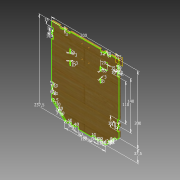
# Autodesk Inventor part: chassi_mdf
Saved by Autodesk Inventor 2014 (Build 180170000, 170)
## iProperties
Created: 2014-11-10
Part Number: chassi_mdf
Material: Generic
Document SubType Name: Modeling
Designer: Gabriel
Density: 1 g/cm^3
Appearance: Default
Author: Gabriel
Autodesk Inventor part; units mm, degrees
ref_plane "YZ Plane" through (0, 0, 0) normal (1, 0, 0) x (0, 1, 0)
ref_plane "XZ Plane" through (0, 0, 0) normal (0, 1, 0) x (-1, 0, 0)
ref_plane "XY Plane" through (0, 0, 0) normal (0, 0, 1) x (1, 0, 0)
sketch "Sketch1" plane through (0, 0, 0) normal (0, 1, 0) x (-1, 0, 0)
  line L0 (40, -237.5) -> (40, -237.5)
  line L1 (40, -237.5) -> (40, -237.5)
  line L2 (0, 0) -> (2.5, 0)
  line L3 (40, -237.5) -> (40, -237.5)
  line L4 (0, -90) -> (0, -80)
  line L5 (0, -70) -> (0, -45)
  line L6 (5, -45) -> (5, -35)
  line L7 (5, -35) -> (0, -35)
  line L8 (0, -35) -> (0, -25)
  line L9 (0, -25) -> (5, -25)
  line L10 (5, -25) -> (5, -15)
  line L11 (5, -15) -> (0, -15)
  line L12 (195, -45) -> (195, -35)
  line L13 (195, -35) -> (200, -35)
  line L14 (195, -25) -> (195, -15)
  line L15 (195, -15) -> (200, -15)
  line L16 (0, 0) -> (25, 0)
  line L17 (25, 0) -> (25, -5)
  line L18 (25, -5) -> (35, -5)
  line L19 (35, -5) -> (35, 0)
  line L20 (45, -5) -> (45, 0)
  line L21 (45, -5) -> (55, -5)
  line L22 (55, -5) -> (55, 0)
  line L23 (200, 0) -> (175, 0)
  line L24 (175, 0) -> (175, -5)
  line L25 (175, -5) -> (165, -5)
  line L26 (165, -5) -> (165, 0)
  line L27 (155, -5) -> (155, 0)
  line L28 (155, -5) -> (145, -5)
  line L29 (145, -5) -> (145, 0)
  line L30 (195, -45) -> (200, -45)
  line L31 (200, -45) -> (195, -45)
  line L32 (0, -45) -> (5, -45)
  line L33 (35, -35) -> (35, -25)
  line L34 (35, -45) -> (55, -45)
  line L35 (55, -45) -> (55, -43.5)
  line L36 (146.5, -45) -> (145, -45)
  line L37 (145, -45) -> (145, -43.5)
  line L38 (55, -85) -> (53.5, -85)
  line L39 (145, -85) -> (146.5, -85)
  line L40 (55, -85) -> (55, -75) construction
  line L41 (56.5, -85) -> (56.5, -75)
  line L42 (53.5, -75) -> (53.5, -85)
  arc A0 (53.5, -85) -> (56.5, -85) centre (55, -85) ccw
  arc A1 (56.5, -75) -> (53.5, -75) centre (55, -75) ccw
  line L43 (145, -85) -> (145, -75) construction
  line L44 (146.5, -85) -> (146.5, -75)
  line L45 (143.5, -75) -> (143.5, -85)
  arc A2 (143.5, -85) -> (146.5, -85) centre (145, -85) ccw
  arc A3 (146.5, -75) -> (143.5, -75) centre (145, -75) ccw
  line L46 (55, -45) -> (55, -55) construction
  line L47 (53.5, -45) -> (53.5, -55)
  line L48 (56.5, -55) -> (56.5, -45)
  arc A4 (56.5, -45) -> (53.5, -45) centre (55, -45) ccw
  arc A5 (53.5, -55) -> (56.5, -55) centre (55, -55) ccw
  line L49 (145, -45) -> (145, -55) construction
  line L50 (143.5, -45) -> (143.5, -55)
  line L51 (146.5, -55) -> (146.5, -45)
  arc A6 (146.5, -45) -> (143.5, -45) centre (145, -45) ccw
  arc A7 (143.5, -55) -> (146.5, -55) centre (145, -55) ccw
  line L52 (0, -185) -> (0, -200)
  line L53 (200, -187.5) -> (200, -200)
  line L54 (200, -187.5) -> (200, -200)
  circle A8 centre (2.5, -170) radius 1.5
  line L55 (0, -138.5) -> (0, -155)
  line L56 (2.5, -175) -> (0, -175)
  line L57 (0, -175) -> (5, -175)
  line L58 (5, -175) -> (5, -185)
  line L59 (5, -185) -> (0, -185)
  line L60 (2.5, -165) -> (0, -165)
  line L61 (2.5, -165) -> (5, -165)
  line L62 (5, -165) -> (5, -155)
  line L63 (5, -155) -> (0, -155)
  line L64 (0, -25) -> (5, -25)
  line L65 (195, -25) -> (200, -25)
  line L66 (0, -25) -> (5, -25)
  line L67 (35, -25) -> (40, -25)
  line L68 (2.5, -35) -> (2.5, -30)
  circle A9 centre (2.5, -30) radius 1.5
  line L69 (40, 0) -> (40, -2.5)
  circle A10 centre (40, -2.5) radius 1.5
  line L70 (160, -1) -> (160, -2.5)
  circle A11 centre (160, -2.5) radius 1.5
  line L71 (197.5, -35) -> (197.5, -30)
  circle A12 centre (197.5, -30) radius 1.5
  line L72 (200, -145) -> (200, -135)
  line L73 (200, -135) -> (200, -145)
  line L74 (200, -135) -> (200, -145)
  line L75 (200, -82.5) -> (200, -90)
  line L76 (200, -100) -> (200, -125)
  line L77 (200, -80) -> (200, -82.5)
  line L78 (200, -82.5) -> (200, -90)
  line L79 (200, -100) -> (200, -125)
  line L80 (0, -120) -> (0, -100)
  line L81 (0, -90) -> (0, -80)
  line L82 (0, -70) -> (0, 0)
  line L83 (0, -175) -> (0, -165)
  line L84 (0, -155) -> (0, -120)
  line L85 (80, -237.5) -> (120, -237.5)
  line L86 (0, 0) -> (25, 0)
  line L87 (35, 0) -> (45, 0)
  line L88 (55, 0) -> (145, 0)
  line L89 (155, 0) -> (165, 0)
  line L90 (175, 0) -> (200, 0)
  line L91 (200, 0) -> (200, -15)
  line L92 (200, -25) -> (200, -35)
  line L93 (200, -45) -> (200, -70)
  line L94 (0, -100) -> (0, -90)
  line L95 (0, -80) -> (0, -70)
  line L96 (200, -100) -> (200, -90)
  line L97 (200, -80) -> (200, -70)
  line L98 (0, -175) -> (0, -165)
  line L99 (0, -155) -> (0, -120)
  line L100 (0, -120) -> (0, -155)
  line L101 (0, -165) -> (0, -175)
  line L102 (0, -175) -> (0, -165)
  line L103 (0, -155) -> (0, -100)
  line L104 (200, -125) -> (200, -135)
  line L105 (200, -145) -> (200, -155)
  circle A13 centre (197.5, -170) radius 1.5
  line L106 (200, -170) -> (200, -165)
  line L107 (200, -165) -> (195, -165)
  line L108 (195, -165) -> (195, -155)
  line L109 (195, -155) -> (200, -155)
  line L110 (200, -170) -> (200, -175)
  line L111 (200, -175) -> (195, -175)
  line L112 (195, -175) -> (195, -185)
  line L113 (195, -185) -> (200, -185)
  line L114 (200, -165) -> (200, -175)
  line L115 (200, -185) -> (200, -187.5)
  line L116 (200, -165) -> (200, -175)
  line L117 (200, -185) -> (200, -187.5)
  line L118 (2.5, -170) -> (4, -170)
  line L119 (40, -237.5) -> (50, -237.5)
  line L120 (60, -237.5) -> (70, -237.5)
  line L121 (40, -237.5) -> (50, -237.5)
  line L122 (50, -237.5) -> (50, -232.5)
  line L123 (50, -232.5) -> (60, -232.5)
  line L124 (60, -232.5) -> (60, -237.5)
  line L125 (60, -237.5) -> (70, -237.5)
  line L126 (70, -237.5) -> (70, -232.5)
  line L127 (70, -232.5) -> (80, -232.5)
  line L128 (80, -232.5) -> (80, -237.5)
  circle A14 centre (65, -235) radius 1.5
  line L129 (160, -237.5) -> (150, -237.5)
  line L130 (150, -237.5) -> (150, -232.5)
  line L131 (150, -232.5) -> (140, -232.5)
  line L132 (140, -232.5) -> (140, -237.5)
  line L133 (140, -237.5) -> (130, -237.5)
  line L134 (130, -237.5) -> (130, -232.5)
  line L135 (130, -232.5) -> (120, -232.5)
  line L136 (120, -232.5) -> (120, -237.5)
  line L137 (130, -237.5) -> (140, -237.5)
  line L138 (150, -237.5) -> (160, -237.5)
  circle A15 centre (135, -235) radius 1.5
  line L139 (40, -237.5) -> (40, -232.5)
  line L140 (160, -237.5) -> (160, -232.5)
  line L141 (195, -204.6875) -> (191.0053, -208.4325)
  line L142 (191.0053, -208.4325) -> (195, -204.6875)
  line L143 (194.9237, -204.759) -> (200, -200)
  line L144 (160, -237.5) -> (169.1192, -228.9507)
  line L145 (169.1192, -228.9507) -> (165.6995, -225.303)
  line L146 (165.6995, -225.303) -> (172.9949, -218.4636)
  line L147 (172.9949, -218.4636) -> (176.4146, -222.1113)
  line L148 (180.2903, -211.6242) -> (183.71, -215.2719)
  line L149 (180.2903, -211.6242) -> (187.5856, -204.7848)
  line L150 (187.5856, -204.7848) -> (191.0053, -208.4325)
  line L151 (176.4146, -222.1113) -> (180.0623, -218.6916)
  line L152 (180.0623, -218.6916) -> (178.3524, -216.8678)
  circle A16 centre (178.3524, -216.8678) radius 1.5
  line L153 (160, -237.5) -> (169.1192, -228.9507)
  line L154 (176.4146, -222.1113) -> (183.71, -215.2719)
  line L155 (191.0053, -208.4325) -> (195, -204.6875)
  line L156 (40, -237.5) -> (30.8808, -228.9507)
  line L157 (30.8808, -228.9507) -> (34.3005, -225.303)
  line L158 (34.3005, -225.303) -> (27.0051, -218.4636)
  line L159 (27.0051, -218.4636) -> (23.5854, -222.1113)
  line L160 (19.7097, -211.6242) -> (16.29, -215.2719)
  line L161 (19.7097, -211.6242) -> (12.4144, -204.7848)
  line L162 (12.4144, -204.7848) -> (8.9947, -208.4325)
  line L163 (23.5854, -222.1113) -> (19.9377, -218.6916)
  line L164 (19.9377, -218.6916) -> (21.6476, -216.8678)
  circle A17 centre (21.6476, -216.8678) radius 1.5
  line L165 (8.9947, -208.4325) -> (0, -200)
  line L166 (40, -237.5) -> (30.8808, -228.9507)
  line L167 (23.5854, -222.1113) -> (16.29, -215.2719)
  line L168 (160, -237.5) -> (200, -200)
  line L169 (200, -200) -> (200, -195)
  line L170 (160, -237.5) -> (156.5803, -233.8523)
  line L171 (156.5803, -233.8523) -> (165.6995, -225.303)
  line L172 (187.5856, -204.7848) -> (196.7048, -196.2356)
  line L173 (196.7048, -196.2356) -> (200, -200)
  line L174 (160, -237.5) -> (160, -230.6463)
  line L175 (200, -200) -> (192.6894, -200)
  point P0 (55, -80)
  point P1 (145, -80)
  point P2 (55, -50)
  point P3 (145, -50)
  dimension "d489" = 3
  dimension "d514" = 3
  dimension "d41" = 2.5
  dimension "d381" = 5
  dimension "d382" = 10
  dimension "d383" = 10
  dimension "d384" = 5
  dimension "d385" = 10
  dimension "d392" = 5
  dimension "d393" = 10
  dimension "d458" = 35
  dimension "d460" = 20
  dimension "d465" = 10
  dimension "d466" = 3
  dimension "d467" = 10
  dimension "d468" = 3
  dimension "d469" = 10
  dimension "d470" = 3
  dimension "d471" = 10
  dimension "d472" = 3
  dimension "d512" = 3
  dimension "d513" = 3
  dimension "d515" = 3
  dimension "d530" = 10
  dimension "d531" = 5
  dimension "d532" = 5
  dimension "d533" = 10
  dimension "d535" = 200
  dimension "d573" = 10
  dimension "d574" = 140
  dimension "d575" = 110
  dimension "d576" = 30
  dimension "d580" = 15
  dimension "d581" = 3
  dimension "d583" = 5
  dimension "d584" = 10
  dimension "d586" = 5
  dimension "d587" = 10
  dimension "d594" = 120
  dimension "d595" = 10
  dimension "d596" = 5
  dimension "d597" = 10
  dimension "d598" = 10
  dimension "d599" = 10
  dimension "d600" = 3
  dimension "d602" = 5
  dimension "d603" = 10
  dimension "d604" = 10
  dimension "d605" = 10
  dimension "d606" = 3
  dimension "d611" = 40
  dimension "d612" = 25
  dimension "d613" = 70
  dimension "d636" = 200
  dimension "d637" = 37.5
  dimension "d638" = 237.5
  dimension "d653" = 5
  dimension "d654" = 10
  dimension "d655" = 10
  dimension "d656" = 10
  dimension "d657" = 5
  dimension "d658" = 2.5
  dimension "d659" = 3
  dimension "d662" = 5
  dimension "d663" = 90
  dimension "d664" = 10
  constraints: 360 end point, 158 perpendicular, 59 parallel, 20 collinear, 18 point on circle, 16 centre point, 16 tangent, 15 point on line, 11 midpoint, 7 coincident, 1 horizontal alignment, 1 vertical alignment, 4 other
  measures "d41" distance of L2.start L2.end
  measures "d381" distance of L6.start L5.end
  measures "d382" distance of L6.start L6.end
  measures "d383" distance of L7.end L8.end
  measures "d384" distance of L8.end L9.end
  measures "d385" distance of L9.end L10.end
  measures "d392" distance of L16.end L17.end
  measures "d393" distance of L17.end L18.end
  measures "d458" distance of L5.end L34.start
  measures "d460" distance of L34.start L34.end
  measures "d465" distance of L38.start L40.end
  measures "d466" diameter of A1
  measures "d467" distance of L39.start L43.end
  measures "d468" diameter of A3
  measures "d469" distance of L34.end L46.end
  measures "d470" diameter of A5
  measures "d471" distance of L36.end L49.end
  measures "d472" diameter of A7
  measures "d512" diameter of A9
  measures "d513" diameter of A10
  measures "d515" diameter of A12
  measures "d530" distance between parallel lines of L65 L15
  measures "d531" distance from line of L71.end L65
  measures "d532" distance from line of L13 L71.end
  measures "d533" distance from line of L30 L71.start
  measures "d535" distance of L52.end point (0, 0)
  measures "d573" distance of L56.start L60.start
  measures "d574" distance of L68.end L118.start
  measures "d575" distance between parallel lines of L32 L63
  measures "d576" distance between parallel lines of L59 L63
  measures "d580" distance between parallel lines of L23 L15
  measures "d581" diameter of A13
  measures "d583" distance of L106.end L107.end
  measures "d584" distance of L107.end L108.end
  measures "d586" distance of L110.end L111.end
  measures "d587" distance of L111.end L112.end
  measures "d594" distance of L129.start L0.end
  measures "d595" distance of L0.end L119.end
  measures "d596" distance of L119.end L122.end
  measures "d597" distance of L122.end L123.end
  measures "d598" distance of L120.start L120.end
  measures "d599" distance of L126.end L127.end
  measures "d600" diameter of A14
  measures "d602" distance of L129.end L130.end
  measures "d603" distance of L130.end L131.end
  measures "d604" distance of L132.end L133.end
  measures "d605" distance of L134.end L135.end
  measures "d606" diameter of A15
  measures "d611" distance between parallel lines of L136 L128
  measures "d612" horizontal distance of A14.centre L0.start
  measures "d613" distance of A15.centre A14.centre
  measures "d636" distance between parallel lines of L91 L82
  measures "d637" distance from line of L85 L52.end
  measures "d638" distance between parallel lines of L129 L88
  measures "d653" distance of L144.end L145.end
  measures "d654" distance of L145.end L146.end
  measures "d655" distance of L146.end L148.start
  measures "d656" distance of L148.start L149.end
  measures "d657" distance of L147.end L151.end
  measures "d658" distance of L151.end L152.end
  measures "d659" diameter of A16
  measures "d662" distance of L156.end L157.end
  measures "d663" angle of L156 L157
  measures "d664" distance of L157.end L158.end
ref_plane "Work Plane2" through (0, 0, 0) normal (0, -1, 0) x (1, 0, 0)
sketch "Sketch2" plane through (0, 0, 0) normal (0, -1, 0) x (1, 0, 0)
  line L0 (-100, -2.5) -> (-100, -12.5)
  line L1 (-100, -12.5) -> (-90, -12.5)
  line L2 (-100, -12.5) -> (-110, -12.5)
  circle A0 centre (-90, -12.5) radius 2.5
  circle A1 centre (-110, -12.5) radius 2.5
  line L3 (-90, -12.5) -> (-90, -52.5)
  line L4 (-90, -52.5) -> (-110, -52.5)
  line L5 (-110, -52.5) -> (-110, -12.5)
  circle A2 centre (-110, -52.5) radius 2.5
  circle A3 centre (-90, -52.5) radius 2.5
  point P0 (-80, -2.5)
  dimension "d326" = 10
  dimension "d327" = 10
  dimension "d328" = 10
  dimension "d329" = 5
  dimension "d330" = 5
  dimension "d475" = 40
  dimension "d476" = 5
  dimension "d477" = 5
  constraints: 12 end point, 4 centre point, 4 coincident, 2 equal length, 2 perpendicular
  measures "d326" distance of L0.start L0.end
  measures "d327" distance of L0.end L1.end
  measures "d328" distance of L0.end L2.end
  measures "d329" diameter of A0
  measures "d330" diameter of A1
  measures "d475" distance of L3.start L3.end
  measures "d476" diameter of A2
  measures "d477" diameter of A3
ref_plane "Work Plane1" through (0, 0, 0) normal (0, -1, 0) x (1, 0, 0)
sketch "Sketch3" plane through (0, 0, 0) normal (0, -1, 0) x (1, 0, 0)
  point P0 (0, 0)
extrude "Extrusion37" add sketch "Sketch1" along normal blind 5 contours L2 L16 L17 L18 L19 L87 L20 L21 L22 L88 L29 L28 L27 L89 L26 L25 L24 L23 L91 L15 L14 L65 L92 L13 L12 L30 L93 L97 L77 L75 L96 L76 L104 L72 L105 L109 L108 L107 L106 L110 L111 L112 L113 L115 L53 L173 L172 L149 L148 L154 L151 L147 L146 L171 L170 L129 L130 L131 L132 L133 L134 L135 L136 L85 L128 L127 L126 L120 L124 L123 L122 L119 L156 L157 L158 L159 L163 L167 L160 L161 L162 L165 L52 L59 L58 L57 L56 L83 L60 L61 L62 L63 L55 L84 L80 L94 L4 L95 L5 L32 L6 L7 L8 L9 L10 L11 L82 | L175 L172 L173 | L143 L141 L150 L172 L175 | L170 L171 L174 L140 | L140 L174 L171 L145 L144 | A16 | A17
extrude "Extrusion38" cut sketch "Sketch2" against normal blind 5 contours A0 L3 L1 | L1 L3 A0 | A1 L5 L2 | L2 L5 A1 | A3 L4 L3 | L3 L4 A3 | A2 L4 L5 | L5 L4 A2
extrude "Extrusion42" cut sketch "Sketch1" along normal blind 5 contours A16 | A17
body "Solid11"
